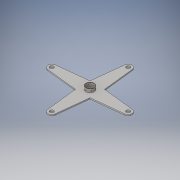
# Autodesk Inventor part: 1-of-4-part holder
Saved by Autodesk Inventor 2016 SP1 (Build 200210100, 210)
## iProperties
Created: 2016-02-22
Part Number: 1-of-4-part holder
Material: Generic
Document SubType Name: Modeling
Designer: Tore Den Store
Density: 1 g/cm^3
Appearance: Default
Author: Tore Den Store
Autodesk Inventor part; units mm, degrees
ref_plane "YZ Plane" through (0, 0, 0) normal (1, 0, 0) x (0, 1, 0)
ref_plane "XY Plane" through (0, 0, 0) normal (0, 0, 1) x (1, 0, 0)
sketch "Sketch1" plane through (0, 0, 0) normal (0, 0, 1) x (1, 0, 0)
  circle A0 centre (0, 0) radius 100
  circle A1 centre (0, 0) radius 110
  dimension "d0" = 200
  dimension "d1" = 10
  constraints: 2 centre point, 1 coincident
  measures "d0" diameter of A0
  measures "d1" radial gap between concentric circles of A0 A1
extrude "Extrusion1" add sketch "Sketch1" along normal blind 200
ref_plane "Work Plane1" through (0, -110, 0) normal (0, 1, 0) x (-1, 0, 0)
sketch "Sketch2" plane through (0, -110, 0) normal (0, 1, 0) x (-1, 0, 0)
  line L0 (110, 200) -> (-110, 200) projected
  line L1 (110, 0) -> (110, 200) projected
  point P0 (0, 0)
  point P1 (0, 150)
  point P2 (0, 50)
  dimension "d4" = 50
  dimension "d5" = 100
  dimension "d6" = 110
  constraints: 1 vertical alignment
  measures "d4" distance from line of L0 point (0, 150)
  measures "d5" distance of point (0, 50) point (0, 150)
  measures "d6" distance from line of L1 point (0, 150)
hole "Hole1" at (0, -110, 150) at (0, -110, 50) direction (0, 1, 0) diameter 8.376 depth 27.3 tip angle 118 counterbore diameter 15 counterbore depth 2 thread size "M10x1.5" class "6H" standard "ANSI Metric M Profile"
pattern_circular "Circular Pattern1" count 6 over 360 about axis through (0, 0, 0) along (0, 0, 1) of "Hole1"
ref_plane "Work Plane2" through (0, 0, 100) normal (0, 0, 1) x (1, 0, 0)
sketch "Sketch3" plane through (0, 0, 100) normal (0, 0, 1) x (1, 0, 0)
  line L0 (0, -212.132) -> (-212.132, 0)
  line L1 (-212.132, 0) -> (0, 212.132)
  line L2 (0, 212.132) -> (212.132, 0)
  line L3 (212.132, 0) -> (0, -212.132)
  line L4 (0, -212.132) -> (0, 212.132) construction
  line L5 (-212.132, 0) -> (212.132, 0) construction
  line L6 (-212.132, 0) -> (-99.384, 1011.0825)
  line L7 (212.132, 0) -> (99.384, 1011.0825)
  arc A0 (99.384, 1011.0825) -> (-99.384, 1011.0825) centre (0, 1000) ccw
  point P0 (0, 0)
  dimension "d18" = 300
  dimension "d22" = 1000
  dimension "d23" = 100
  constraints: 16 end point, 2 equal length, 2 midpoint, 2 parallel, 2 point on circle, 2 tangent, 1 centre point, 1 perpendicular, 1 vertical
  measures "d18" distance of L1.end L2.end
  measures "d22" distance from line of L5 A0.centre
  measures "d23" radius of A0
extrude "Extrusion2" add sketch "Sketch3" along normal mid plane 30
pattern_circular "Circular Pattern2" count 4 over 360 about axis through (0, 0, 0) along (0, 0, 1) of "Extrusion2"
sketch "Sketch4" plane through (0, 0, 115) normal (0, 0, 1) x (1, 0, 0)
  arc A0 (-1011.0825, 99.384) -> (-1011.0825, -99.384) centre (-1000, 0) ccw projected
  arc A1 (99.384, 1011.0825) -> (-99.384, 1011.0825) centre (0, 1000) ccw projected
  arc A2 (1011.0825, -99.384) -> (1011.0825, 99.384) centre (1000, 0) ccw projected
  arc A3 (-99.384, -1011.0825) -> (99.384, -1011.0825) centre (0, -1000) ccw projected
  point P0 (0, 0)
  constraints: 4 coincident
hole "Hole2" at (-1000, 0, 115) at (0, 1000, 115) at (1000, 0, 115) at (0, -1000, 115) direction (0, 0, -1) diameter 100 end through all
sketch "Sketch5" plane through (0, 0, 115) normal (0, 0, 1) x (1, 0, 0)
  circle A0 centre (0, 0) radius 100 projected
extrude "Extrusion3" cut sketch "Sketch5" against normal through all
body "Solid1"
